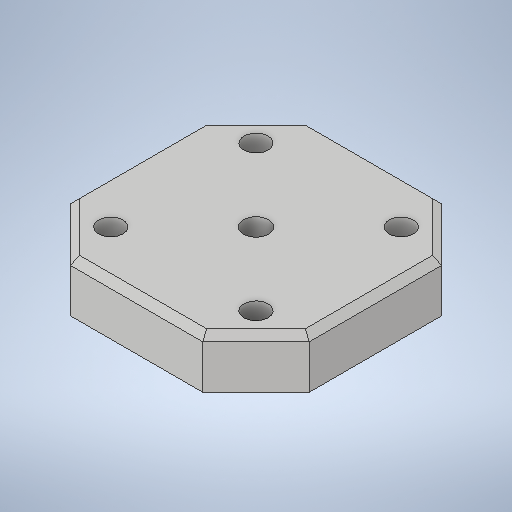
# Autodesk Inventor part: Platform A
Saved by Autodesk Inventor 2025 (Build 290162000, 162)
## iProperties
Created: 2021-01-07
Part Number: Platform A
Material: Generic
Document SubType Name: Modeling
Designer: caleb
Density: 1 g/cm^3
Appearance: Default
Author: caleb
Autodesk Inventor part; units mm, degrees
ref_plane "YZ Plane" through (0, 0, 0) normal (1, 0, 0) x (0, 1, 0)
ref_plane "XZ Plane" through (0, 0, 0) normal (0, 1, 0) x (-1, 0, 0)
ref_plane "XY Plane" through (0, 0, 0) normal (0, 0, 1) x (1, 0, 0)
sketch "Sketch1" plane through (0, 0, 0) normal (0, 1, 0) x (-1, 0, 0)
  line L0 (-14.25, 14.25) -> (14.25, 14.25)
  line L1 (14.25, 14.25) -> (14.25, -14.25)
  line L2 (14.25, -14.25) -> (-14.25, -14.25)
  line L3 (-14.25, -14.25) -> (-14.25, 14.25)
  line L4 (-14.25, 14.25) -> (14.25, -14.25) construction
  line L5 (14.25, 14.25) -> (-14.25, -14.25) construction
  point P0 (0, 0)
  dimension "d0" = 28.5
  dimension "d1" = 28.5
  constraints: 12 end point, 2 midpoint, 2 parallel, 1 horizontal, 1 perpendicular
  measures "d0" distance of L0.end L1.end
  measures "d1" distance of L0.start L0.end
extrude "Extrusion1" add sketch "Sketch1" along normal blind 6
sketch "Sketch2" plane through (0, 6, 0) normal (0, 1, 0) x (1, 0, 0)
  circle A0 centre (0, 0) radius 12.25
  line L0 (-14.25, 14.25) -> (-14.25, -14.25) projected
  line L1 (14.25, -14.25) -> (14.25, 14.25) projected
  line L2 (14.25, 14.25) -> (-14.25, 14.25) projected
  line L3 (0, 0) -> (-8.6621, -8.6621) construction
  line L4 (-8.6621, -8.6621) -> (0.3214, -8.6621) construction
  point P0 (8.6621, -8.6621)
  point P1 (8.6621, 8.6621)
  point P2 (-8.6621, 8.6621)
  dimension "d60" = 24.5
  dimension "d61" = 28.5
  dimension "d62" = 14.25
  dimension "d63" = 28.5
  dimension "d64" = 14.25
  dimension "d69" = 45
  dimension "d72" = 360
  constraints: 4 end point, 1 coincident, 1 horizontal, 8 other
  measures "d61" distance between parallel lines of L0 L1
  measures "d62" distance from line of L0 L3.start
  measures "d63" distance of L0.start L0.end
  measures "d64" distance from line of L2 L3.start
  measures "d69" angle of L4 L3
hole "Hole1" at (8.6621, 6, 8.6621) at (8.6621, 6, -8.6621) at (-8.6621, 6, -8.6621) at (-8.6621, 6, 8.6621) direction (0, -1, 0) diameter 2.9 end through all clearance for "Flat Head Machine Screw" size "M2.5" standard "Ansi Metric M Profile"
sketch "Sketch3" plane through (0, 6, 0) normal (0, 1, 0) x (1, 0, 0)
  circle A0 centre (0, 0) radius 1.4986
  dimension "d22" = 2.9972
  constraints: 1 centre point, 1 coincident
  measures "d22" diameter of A0
extrude "Extrusion2" cut sketch "Sketch3" against normal through all
sketch "Sketch4" plane through (0, 0, 0) normal (0, -1, 0) x (1, 0, 0)
  line L0 (-7.1437, -1.3748) -> (2.3813, -6.8739)
  line L1 (4.7625, -5.4991) -> (4.7625, 5.4991)
  line L2 (2.3813, 6.8739) -> (-7.1437, 1.3748)
  arc A0 (4.7625, 5.4991) -> (2.3813, 6.8739) centre (3.175, 5.4991) ccw
  arc A1 (-7.1437, 1.3748) -> (-7.1437, -1.3748) centre (-6.35, 0) ccw
  arc A2 (2.3813, -6.8739) -> (4.7625, -5.4991) centre (3.175, -5.4991) ccw
  circle A3 centre (0, 0) radius 1.4986 projected
  dimension "d42" = 1.5875
  dimension "d45" = 6.35
  dimension "d57" = 3.175
  dimension "d58" = 5.4991
  dimension "d59" = 5.4991
  constraints: 6 end point, 6 point on circle, 6 tangent, 3 centre point, 2 equal radius, 1 horizontal alignment, 1 vertical
  measures "d42" radius of A0
  measures "d45" distance of A3.centre A1.centre
  measures "d57" horizontal distance of A3.centre A2.centre
  measures "d58" vertical distance of A3.centre A2.centre
  measures "d59" vertical distance of A3.centre A0.centre
extrude "Extrusion3" cut sketch "Sketch4" against normal blind 1.4986
chamfer "Chamfer3" distance 6.35 angle 45 4 edges at (14.25, 3, -14.25) (-14.25, 3, -14.25) (-14.25, 3, 14.25) (14.25, 3, 14.25)
chamfer "Chamfer4" distance 0.7937 angle 45 8 edges at (11.075, 6, -11.075) (0, 6, -14.25) (-11.075, 6, -11.075) (-14.25, 6, 0) (-11.075, 6, 11.075) (0, 6, 14.25) (11.075, 6, 11.075) (14.25, 6, 0)
equation "\"d62\" = 0.5 * d61"
equation "\"d64\" = 0.5 * d63"
equation "\"d59\" = d58"
body "Solid1"
